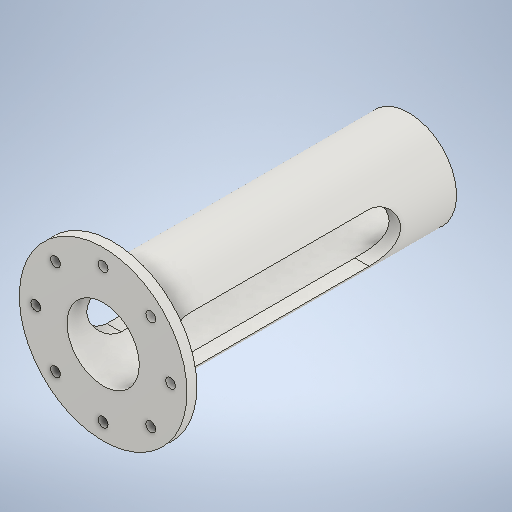
# Autodesk Inventor part: 11 CROSSHEAD GUIDE
Saved by Autodesk Inventor 2025.2 (Build 292293000, 293)
## iProperties
Created: 2025-05-29
Part Number: 11 CROSSHEAD GUIDE
Material: Steel AISI 1020 107 HR
Document SubType Name: Modeling
Designer: bless
Density: 7.87 g/cm^3
Appearance: Steel
Author: bless
Autodesk Inventor part; units mm, degrees
ref_plane "YZ Plane" through (0, 0, 0) normal (1, 0, 0) x (0, 1, 0)
ref_plane "XZ Plane" through (0, 0, 0) normal (0, 1, 0) x (-1, 0, 0)
ref_plane "XY Plane" through (0, 0, 0) normal (0, 0, 1) x (1, 0, 0)
sketch "Sketch1" plane through (0, 0, 0) normal (0, 0, 1) x (1, 0, 0)
  circle A0 centre (0, 0) radius 25.5
  dimension "d0" = 51
  constraints: 1 centre point, 1 coincident
  measures "d0" diameter of A0
extrude "Extrusion1" add sketch "Sketch1" along normal blind 3
sketch "Sketch2" plane through (0, 0, 0) normal (0, 0, -1) x (-1, 0, 0)
  circle A0 centre (0, 0) radius 25.5 projected
  circle A1 centre (0, 0) radius 14.5
  dimension "d3" = 29
  constraints: 1 centre point, 1 coincident
  measures "d3" diameter of A1
extrude "Extrusion2" add sketch "Sketch2" along normal blind 90 contours A1
sketch "Sketch3" plane through (0, 0, 3) normal (0, 0, 1) x (1, 0, 0)
  circle A0 centre (0, 0) radius 25.5 projected
  circle A1 centre (0, 0) radius 20.5
  circle A2 centre (0, 20.5) radius 1.5
  circle A3 centre (-14.4957, 14.4957) radius 1.5
  circle A4 centre (-20.5, 0) radius 1.5
  circle A5 centre (-14.4957, -14.4957) radius 1.5
  circle A6 centre (0, -20.5) radius 1.5
  circle A7 centre (14.4957, -14.4957) radius 1.5
  circle A8 centre (20.5, 0) radius 1.5
  circle A9 centre (14.4957, 14.4957) radius 1.5
  dimension "d6" = 41
  dimension "d7" = 3
  dimension "d10" = 360
  constraints: 8 centre point, 2 vertical alignment, 1 coincident, 19 other
  measures "d7" diameter of A2
extrude "Extrusion3" cut sketch "Sketch3" against normal through all contours A1 A8 | A1 A8 | A9 A1 | A1 A9 | A7 A1 | A1 A7 | A2 A1 | A1 A2 | A6 A1 | A1 A6 | A3 A1 | A1 A3 | A5 A1 | A1 A5 | A4 A1 | A1 A4
sketch "Sketch4" plane through (0, 0, 3) normal (0, 0, 1) x (1, 0, 0)
  circle A0 centre (0, 0) radius 25.5 projected
  circle A1 centre (0, 0) radius 11
  dimension "d14" = 22
  constraints: 1 centre point, 1 coincident
  measures "d14" diameter of A1
extrude "Extrusion4" cut sketch "Sketch4" against normal through all contours A1
sketch "Sketch5" plane through (0, 0, 0) normal (1, 0, 0) x (0, 1, 0)
  line L0 (0, -10.5) -> (0, -65.5)
  arc A0 (-7.5, -65.5) -> (7.5, -65.5) centre (0, -65.5) ccw
  arc A1 (7.5, -10.5) -> (-7.5, -10.5) centre (0, -10.5) ccw
  line L1 (7.5, -10.5) -> (7.5, -65.5)
  line L2 (-7.5, -65.5) -> (-7.5, -10.5)
  line L3 (25.5, 3) -> (-25.5, 3) projected
  point P0 (0, 0)
  point P1 (0, -3)
  point P2 (0, 3)
  dimension "d17" = 7.5
  dimension "d18" = 7.5
  dimension "d22" = 55
  dimension "d23" = 13.5
  constraints: 6 end point, 5 point on circle, 3 tangent, 2 centre point, 2 coincident, 1 midpoint, 1 vertical
  measures "d17" radius of A0
  measures "d18" radius of A1
  measures "d22" distance of L0.end L0.start
  measures "d23" distance of point (0, 3) L0.start
extrude "Extrusion5" cut sketch "Sketch5" along normal through all both and the other way through all
body "Solid1"
